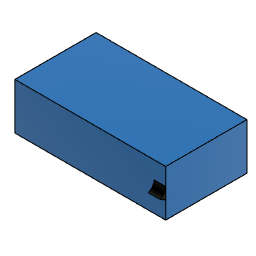
Powerstack v5 (Autodesk Fusion 360 archive; units mm, degrees)
design "Backup Battery"
Autodesk Fusion 360 part; units mm, degrees
sketch "Sketch1" plane through (0, 0, 0) normal (0, 0, 1) x (1, 0, 0)
  line L0 (0, 0) -> (130, 0)
  line L1 (130, 0) -> (130, 70)
  line L2 (130, 70) -> (0, 70)
  line L3 (0, 70) -> (0, 0)
  dimension "d1" = 130
  dimension "d2" = 70
  constraint horizontal L0
  constraint vertical L1
  constraint horizontal L2
  constraint vertical L3
  constraint coincident L0.start L3.end
  measures "d1" distance of L0.start L0.end
  measures "d2" distance of L0.start L2.end
extrude "Extrude1" add sketch "Sketch1" along normal blind 40 makes body 1
sketch "Sketch2" plane through (130, 0, 0) normal (1, 0, 0) x (0, 1, 0)
  line L0 (0, 0) -> (70, 0)
  line L1 (70, 0) -> (70, 40)
  line L2 (70, 40) -> (0, 40)
  line L3 (0, 40) -> (0, 0)
  arc A0 (-5, 18) -> (0, 25) centre (-7.4, 25) ccw
  line L4 (-5, 18) -> (0, 15)
  constraint tangent L3 A0
  constraint coincident L3 A0.end
  constraint coincident L3 L4.end
extrude "Extrude2" add sketch "Sketch2" against normal blind 10 separate body contours L3 A0 L4 makes body 2

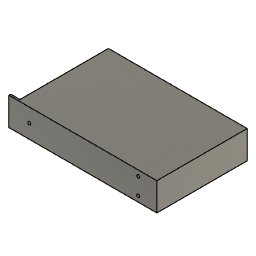
design "Powerbrick"
Autodesk Fusion 360 part; units mm, degrees
sketch "Sketch1" plane through (0, 0, 0) normal (0, 0, 1) x (1, 0, 0)
  line L0 (0, 0) -> (159, 0)
  line L1 (159, 0) -> (159, 97)
  line L2 (159, 97) -> (0, 97)
  line L3 (0, 97) -> (0, 0)
  dimension "d1" = 159
  dimension "d2" = 97
  constraint horizontal L0
  constraint vertical L1
  constraint horizontal L2
  constraint vertical L3
  constraint coincident L0.start L3.end
  measures "d1" distance of L0.start L0.end
  measures "d2" distance of L0.start L2.end
extrude "Extrude1" add sketch "Sketch1" along normal blind 30
sketch "Sketch2" plane through (0, 0, 30) normal (0, 0, 1) x (-1, 0, 0)
  line L0 (0, -97) -> (0, 0)
  line L1 (0, 0) -> (-159, 0)
  line L2 (-159, 0) -> (-159, -97)
  line L3 (-159, -97) -> (0, -97)
  line L4 (0, -97) -> (-10, -97)
  line L5 (-10, -97) -> (-10, -2)
  line L6 (-10, -2) -> (0, -2)
  line L7 (0, -2) -> (0, -97)
  dimension "d5" = 10
  dimension "d6" = 95
  constraint horizontal L4
  constraint vertical L5
  constraint horizontal L6
  constraint vertical L7
  constraint coincident L0.start L3.end
  measures "d5" distance of L0.start L4.end
  measures "d6" distance of L0.start L6.end
extrude "Extrude2" cut sketch "Sketch2" against normal blind 28 contours L0 L3 L4 L5 L6 L7
sketch "Sketch3" plane through (0, 0, 0) normal (0, -1, 0) x (1, 0, 0)
  line L0 (0, 0) -> (159, 0)
  line L1 (159, 0) -> (159, 30)
  line L2 (159, 30) -> (0, 30)
  line L3 (0, 30) -> (0, 0)
  line L4 (0, 0) -> (22, 0) construction
  line L5 (22, 0) -> (22, 15) construction
  line L6 (22, 15) -> (0, 15) construction
  line L7 (0, 15) -> (0, 0) construction
  line L8 (139, 0) -> (139, 30) construction
  circle A0 centre (139, 6) radius 1.6
  circle A1 centre (139, 24) radius 1.6
  circle A2 centre (22, 15) radius 1.6
  dimension "d9" = 22
  dimension "d10" = 15
  dimension "d11" = 117
  dimension "d12" = 3.2
  dimension "d13" = 6
  dimension "d14" = 18
  constraint horizontal L4
  constraint vertical L5
  constraint horizontal L6
  constraint vertical L7
  constraint coincident L0.start L3.end
  constraint coincident L0 L8.start
  constraint coincident L2 L8.end
  constraint perpendicular L2 L8
  constraint coincident L8 A0.centre
  constraint coincident L8 A1.centre
  constraint coincident L5.end L6.start
  constraint equal A1 A2
  constraint equal A0 A1
  measures "d9" distance of L0.start L4.end
  measures "d10" distance of L0.start L6.end
  measures "d11" distance of L5 L8
  measures "d12" diameter of A1
  measures "d13" distance of L0 A0.centre
  measures "d14" distance of A0.centre A1.centre
extrude "Extrude3" cut sketch "Sketch3" against normal blind 10 contours A0 | A1 | A2
